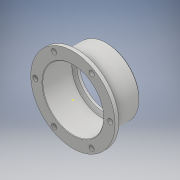
# Autodesk Inventor part: Деталь3
Saved by Autodesk Inventor 2018.1 (Build 221171000, 171)
## iProperties
Created: 2023-05-15
Part Number: Деталь3
Material: Типовые
Document SubType Name: Modeling
Designer: student
Density: 1 g/cm^3
Appearance: По умолчанию
Author: student
Autodesk Inventor part; units mm, degrees
ref_plane "YZ Plane" through (0, 0, 0) normal (1, 0, 0) x (0, 1, 0)
ref_plane "XZ Plane" through (0, 0, 0) normal (0, 1, 0) x (-1, 0, 0)
ref_plane "XY Plane" through (0, 0, 0) normal (0, 0, 1) x (1, 0, 0)
sketch "Эскиз1" plane through (0, 0, 0) normal (0, 1, 0) x (-1, 0, 0)
  circle A0 centre (0, 0) radius 90
  dimension "d0" = 180
  constraints: 1 centre point, 1 coincident
  measures "d0" diameter of A0
extrude "Выдавливание1" add sketch "Эскиз1" along normal blind 8
sketch "Эскиз2" plane through (0, 8, 0) normal (0, 1, 0) x (1, 0, 0)
  circle A0 centre (0, 0) radius 70
  dimension "d3" = 140
  constraints: 1 centre point, 1 coincident
  measures "d3" diameter of A0
extrude "Выдавливание2" add sketch "Эскиз2" along normal blind 65
hole "Отверстие1" at (-1.069, 73, 0) direction (0, -1, 0) diameter 115 depth 10 tip angle 118
hole "Отверстие2" at (-0.208, 0, -0.4159) direction (0, 1, 0) diameter 130 depth 63 tip angle 118
chamfer "Фаска1" distance 2 angle 45 1 edges at (-70, 73, 0)
chamfer "Фаска2" distance 1 angle 45 1 edges at (-0.208, 0, 64.5841)
sketch "Эскиз3" plane through (0, 8, 0) normal (0, 1, 0) x (1, 0, 0)
  circle A0 centre (0, 0) radius 80
  circle A1 centre (80, 0) radius 5.5
  circle A2 centre (40, -69.282) radius 5.5
  circle A3 centre (-40, -69.282) radius 5.5
  circle A4 centre (-80, 0) radius 5.5
  circle A5 centre (-40, 69.282) radius 5.5
  circle A6 centre (40, 69.282) radius 5.5
  dimension "d30" = 160
  dimension "d31" = 11
  dimension "d34" = 360
  constraints: 6 centre point, 1 coincident, 1 horizontal alignment, 15 other
  measures "d31" diameter of A1
extrude "Выдавливание3" cut sketch "Эскиз3" against normal blind 100 contours A0 A1 | A0 A1 | A6 A0 | A0 A6 | A2 A0 | A0 A2 | A5 A0 | A0 A5 | A3 A0 | A0 A3 | A4 A0 | A0 A4
sketch "Эскиз4" plane through (0, 0, 0) normal (0, -1, 0) x (1, 0, 0)
  point P0 (0, 0)
